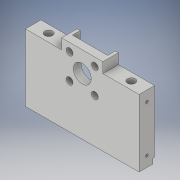
# Autodesk Inventor part: back mount
Saved by Autodesk Inventor 2017 (Build 210142000, 142)
## iProperties
Created: 2016-07-18
Part Number: back mount
Material: Generic
Document SubType Name: Modeling
Designer: Darien Morrow
Density: 1 g/cm^3
Appearance: Default
Author: Darien Morrow
Autodesk Inventor part; units mm, degrees
ref_plane "YZ Plane" through (0, 0, 0) normal (1, 0, 0) x (0, 1, 0)
ref_plane "XZ Plane" through (0, 0, 0) normal (0, 1, 0) x (-1, 0, 0)
ref_plane "XY Plane" through (0, 0, 0) normal (0, 0, 1) x (1, 0, 0)
sketch "Sketch1" plane through (0, 0, 0) normal (0, 0, 1) x (1, 0, 0)
  line L0 (0, 0) -> (139.7, 0)
  line L1 (139.7, 0) -> (139.7, 82.55)
  line L2 (139.7, 82.55) -> (0, 82.55)
  line L3 (0, 82.55) -> (0, 0)
  line L4 (95.25, 82.55) -> (44.45, 82.55)
  line L5 (44.45, 82.55) -> (44.45, 95.25)
  line L6 (44.45, 95.25) -> (95.25, 95.25)
  line L7 (95.25, 95.25) -> (95.25, 82.55)
  point P0 (69.85, 82.55)
  dimension "d0" = 139.7
  dimension "d1" = 82.55
  dimension "d2" = 12.7
  dimension "d3" = 50.8
  dimension "d4" = 25.4
  dimension "d62" = 69.85
  constraints: 16 end point, 4 parallel, 2 horizontal, 2 perpendicular, 1 midpoint, 1 point on line
  measures "d0" distance between parallel lines of L1 L3
  measures "d1" distance between parallel lines of L0 L2
  measures "d2" distance between parallel lines of L2 L6
  measures "d3" distance between parallel lines of L5 L7
  measures "d4" distance from line of point (69.85, 82.55) L7
  measures "d62" distance from line of point (69.85, 82.55) L1
extrude "Extrusion1" add sketch "Sketch1" along normal blind 19.05
sketch "Sketch2" plane through (0, 0, 0) normal (0, 0, -1) x (-1, 0, 0)
  line L0 (-44.45, 82.55) -> (0, 82.55) projected
  line L1 (-139.7, 0) -> (-139.7, 82.55) projected
  point P0 (0, 0)
  point P1 (-69.85, 69.85)
  dimension "d7" = 12.7
  dimension "d8" = 69.85
  measures "d7" distance from line of point (-69.85, 69.85) L0
  measures "d8" distance from line of L1 point (-69.85, 69.85)
hole "Hole1" at (69.85, 69.85, 0) direction (0, 0, 1) diameter 22 depth 25.4 tip angle 118
sketch "Sketch3" plane through (0, 0, 0) normal (0, 0, -1) x (-1, 0, 0)
  line L0 (-91.44, 48.26) -> (-48.26, 48.26)
  line L1 (-48.26, 48.26) -> (-48.26, 91.44)
  line L2 (-48.26, 91.44) -> (-91.44, 91.44)
  line L3 (-91.44, 91.44) -> (-91.44, 48.26)
  line L4 (-91.44, 48.26) -> (-48.26, 91.44) construction
  line L5 (-48.26, 48.26) -> (-91.44, 91.44) construction
  line L6 (-44.45, 82.55) -> (0, 82.55) projected
  line L7 (-95.25, 95.25) -> (-44.45, 95.25) projected
  line L8 (-91.44, 91.44) -> (-48.26, 91.44)
  line L9 (-48.26, 91.44) -> (-48.26, 95.25)
  line L10 (-48.26, 95.25) -> (-91.44, 95.25)
  line L11 (-91.44, 95.25) -> (-91.44, 91.44)
  line L12 (-139.7, 0) -> (-139.7, 82.55) projected
  point P0 (0, 0)
  point P1 (-69.85, 69.85)
  dimension "d16" = 12.7
  dimension "d17" = 43.18
  dimension "d18" = 43.18
  dimension "d21" = 69.85
  dimension "d22" = 43.18
  constraints: 20 end point, 4 parallel, 2 horizontal, 2 midpoint, 2 perpendicular, 1 point on line
  measures "d16" distance from line of L6 point (-69.85, 69.85)
  measures "d17" distance between parallel lines of L0 L2
  measures "d18" distance between parallel lines of L1 L3
  measures "d21" distance from line of point (-69.85, 69.85) L12
  measures "d22" distance between parallel lines of L9 L11
extrude "Extrusion2" cut sketch "Sketch3" against normal blind 9.525
sketch "Sketch4" plane through (0, 0, 19.05) normal (0, 0, 1) x (1, 0, 0)
  line L0 (54.35, 54.35) -> (85.35, 54.35)
  line L1 (85.35, 54.35) -> (85.35, 85.35)
  line L2 (85.35, 85.35) -> (54.35, 85.35)
  line L3 (54.35, 85.35) -> (54.35, 54.35)
  line L4 (54.35, 54.35) -> (85.35, 85.35) construction
  line L5 (85.35, 54.35) -> (54.35, 85.35) construction
  line L6 (139.7, 82.55) -> (95.25, 82.55) projected
  line L7 (139.7, 0) -> (139.7, 82.55) projected
  point P0 (0, 0)
  point P1 (69.85, 69.85)
  dimension "d23" = 12.7
  dimension "d24" = 69.85
  dimension "d25" = 31
  dimension "d26" = 31
  constraints: 12 end point, 4 coincident, 2 midpoint, 2 parallel, 1 horizontal, 1 perpendicular
  measures "d23" distance from line of L6 point (69.85, 69.85)
  measures "d24" distance from line of L7 point (69.85, 69.85)
  measures "d25" distance between parallel lines of L1 L3
  measures "d26" distance between parallel lines of L0 L2
hole "Hole2" at (54.35, 85.35, 19.05) at (54.35, 54.35, 19.05) at (85.35, 85.35, 19.05) at (85.35, 54.35, 19.05) direction (0, 0, -1) diameter 3.4036 end through all counterbore diameter 8.4074 counterbore depth 5.715 clearance for "Hex Head Machine Screw" size "M3" standard "Ansi Metric M Profile"
sketch "Sketch5" plane through (0, 0, 0) normal (0, -1, 0) x (1, 0, 0)
  line L0 (120.65, 9.525) -> (19.05, 9.525)
  line L1 (0, 0) -> (139.7, 0) projected
  line L2 (139.7, 0) -> (139.7, 19.05) projected
  dimension "d34" = 101.6
  dimension "d35" = 9.525
  dimension "d36" = 19.05
  constraints: 2 coincident, 2 end point, 1 horizontal
  measures "d34" distance of L0.end L0.start
  measures "d35" distance between parallel lines of L0 L1
  measures "d36" distance from line of L0.start L2
hole "Hole3" at (120.65, 0, 9.525) at (19.05, 0, 9.525) direction (0, 1, 0) diameter 9.6012 end through all
sketch "Sketch6" plane through (0, 0, 0) normal (0, 0, -1) x (-1, 0, 0)
  line L0 (-120.65, 28.575) -> (-19.05, 28.575)
  line L1 (-44.45, 82.55) -> (0, 82.55) projected
  line L2 (0, 82.55) -> (0, 0) projected
  dimension "d44" = 101.6
  dimension "d45" = 53.975
  dimension "d46" = 19.05
  constraints: 2 coincident, 2 end point, 1 horizontal
  measures "d44" distance of L0.end L0.start
  measures "d45" distance between parallel lines of L0 L1
  measures "d46" distance from line of L0.end L2
hole "Hole4" at (120.65, 28.575, 0) at (19.05, 28.575, 0) direction (0, 0, 1) diameter 3.302 depth 12.2936 tip angle 118 thread size "8-32 UNC" class "2B" standard "ANSI Unified Screw Threads"
sketch "Sketch7" plane through (0, 0, 0) normal (-1, 0, 0) x (0, 0, 1)
  line L0 (9.525, 95.25) -> (9.525, 48.26) projected
  line L1 (9.525, 69.055) -> (9.525, 11.905)
  point P0 (0, 0)
  point P1 (9.525, 89.85)
  dimension "d54" = 57.15
  constraints: 2 coincident, 2 end point, 1 collinear, 1 point on line
  measures "d54" distance of L1.end L1.start
hole "Hole5" at (0, 69.055, 9.525) at (0, 11.905, 9.525) direction (1, 0, 0) diameter 3.302 depth 12.2936 tip angle 118 thread size "8-32 UNC" class "2B" standard "ANSI Unified Screw Threads"
sketch "Sketch8" plane through (139.7, 0, 0) normal (1, 0, 0) x (0, 0, -1)
  line L0 (-19.05, 82.55) -> (-19.05, 0) projected
  line L1 (0, 0) -> (-19.05, 0) projected
  point P0 (-9.525, 12.7)
  point P1 (-9.525, 69.85)
  dimension "d87" = 57.15
  dimension "d88" = 9.525
  dimension "d89" = 9.525
  dimension "d90" = 12.7
  measures "d87" distance of point (-9.525, 69.85) point (-9.525, 12.7)
  measures "d88" distance from line of L0 point (-9.525, 12.7)
  measures "d89" distance from line of L0 point (-9.525, 69.85)
  measures "d90" distance from line of point (-9.525, 12.7) L1
sketch "Sketch9" plane through (0, 0, 0) normal (0, 0, -1) x (-1, 0, 0)
  line L0 (-139.7, 41.275) -> (0, 41.275)
  line L1 (0, 0) -> (-139.7, 0) projected
  line L2 (-101.6, 31.369) -> (-38.1, 31.369)
  line L3 (0, 82.55) -> (0, 0) projected
  line L4 (-44.45, 82.55) -> (0, 82.55) projected
  line L5 (0, 82.55) -> (-31.75, 41.275)
  line L6 (-17.1517, 76.4998) -> (-38.7838, 52.9606)
  point P0 (-27.3538, 68.7266)
  dimension "d63" = 41.275
  dimension "d64" = 9.906
  dimension "d65" = 139.7
  dimension "d66" = 0
  dimension "d67" = 31.75
  dimension "d68" = 9.906
  dimension "d69" = 12.7
  dimension "d71" = 63.5
  dimension "d72" = 38.1
  dimension "d101" = 11.43
  constraints: 8 end point, 2 coincident, 2 horizontal, 1 point on line
  measures "d63" distance between parallel lines of L0 L1
  measures "d64" distance between parallel lines of L2 L0
  measures "d65" distance of L0.end L0.start
  measures "d66" distance from line of L0.end L3
  measures "d67" distance of L0.end L5.end
  measures "d68" distance from line of L5 L6.start
  measures "d69" distance from line of L5 L6.end
  measures "d71" distance of L2.end L2.start
  measures "d72" distance from line of L3 L2.end
  measures "d101" horizontal distance of point (-27.354, 68.727) L6.end
hole "Hole6" at (27.3538, 68.7266, 0) at (38.1, 31.369, 0) at (101.6, 31.369, 0) direction (0, 0, 1) diameter 3.302 depth 12.2936 tip angle 118 thread size "8-32 UNC" class "2B" standard "ANSI Unified Screw Threads"
hole "Hole8" at (139.7, 12.7, 9.525) at (139.7, 69.85, 9.525) direction (-1, 0, 0) diameter 3.302 depth 12.2936 tip angle 118 thread size "8-32 UNC" class "2B" standard "ANSI Unified Screw Threads"
sketch "Sketch10" plane through (0, 0, 0) normal (0, -1, 0) x (1, 0, 0)
  point P0 (0, 0)
sketch "Sketch11" plane through (0, 0, 0) normal (0, -1, 0) x (1, 0, 0)
  line L0 (139.7, 0) -> (95.25, 0) projected
  line L1 (0, 0) -> (0, 19.05) projected
  line L2 (139.7, 0) -> (0, 0)
  line L3 (0, 0) -> (0, 2.032)
  line L4 (0, 2.032) -> (139.7, 2.032)
  line L5 (139.7, 2.032) -> (139.7, 0)
  dimension "d98" = 2.032
  constraints: 8 end point, 2 parallel, 1 horizontal, 1 perpendicular, 1 point on line
  measures "d98" distance between parallel lines of L4 L2
extrude "Extrusion3" cut sketch "Sketch11" against normal blind 6.35
body "Solid1"
